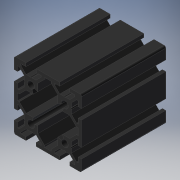
# Autodesk Inventor part: HFS5-4040-50
Saved by Autodesk Inventor 2019 (Build 230136000, 136)
## iProperties
Created: 2023-10-13
Part Number: HFS5-4040-50
Material: Generic
Catalog Web Link: www.cadenas.de
Description: NFS5-4040, NFSB5-4040, HFS5-4040, HFSB5-4040, CAF5-4040, NFSF5-4040, HFSF5-4040, HFST5-4040, HFSY5-4040-Aluminum Frames -5 Series-2 Row Groove 40 mm Square-Specified Length
Vendor: MISUMI
Document SubType Name: Modeling
Designer: psAdmin
Manufacturer: MISUMI
Mass: 24.0436 g
Surface Area: 253.98 cm^2
Volume: 24.0436 cm^3
Density: 1 g/cm^3
Appearance: PSOLRGB-175-175-175
Category: PARTsolutions
Company: MISUMI
Title: HFS5-4040-50
Author: Cadenas PARTsolutions
Comments: Aluminum Frames -5 Series-2 Row Groove 40 mm Square-Specified Length
PSOL_IDENT_0: {$CADENAS_DATA/23d-libs/misumi/metric/38_al_extrusions_blackets/5/hfs5_4040.prj},637 {VTYP=3D},{NB=H
PSOL_IDENT_1: FS5-4040-50},{LINA=HFS5-4040-50},{NN=NFS5-4040, NFSB5-4040, HFS5-4040, HFSB5-4040, CAF5-4040, NFSF5-
PSOL_IDENT_2: 4040, HFSF5-4040, HFST5-4040, HFSY5-4040},{DATE=08.05.2023 08:46:43},{GEOMDATE=23.09.2021 06:48:02},
PSOL_IDENT_3: {VERSION=},{LINEID=150},{WBVAR=L,ALT1,ALT2,ALT4,ALT5,CP5,DL5,DR5,ALT6,ALT9,ALT10,ALT11,HP6,NHL6,DL6,
PSOL_IDENT_4: NHR6,DR6,ALT7,ALT8,NH9,AH,BH,CH,DH,EH,NH10,AV,BV,CV,DV,EV,NH11,AP,BP,CP,DP,EP,ALT12,ALT13,Z,NH12,XA,
PSOL_IDENT_5: XB,XC,XD,XE,NH13,YA,YB,YC,YD,YE,ALT16,HP16,DL16,DR16,ALT17,HQ17,JLP,ALT18,HQ18,KLP,ALT20},{WBNUMERIC=
PSOL_IDENT_6: L,NH9,AH,BH,CH,DH,EH,NH10,AV,BV,CV,DV,EV,NH11,AP,BP,CP,DP,EP,NH12,XA,XB,XC,XD,XE,NH13,YA,YB,YC,YD,YE
PSOL_IDENT_7: ,HQ17,JLP,HQ18,KLP}  {NB=HFS5-4040-50},{LINA=HFS5-4040-50},{KT=DUMMY},{PN=HFS5-4040-50},{TPS=HFS5-40
PSOL_IDENT_8: 40},{MAT=A6N01SS-T5 Aluminum Alloy or 6005A-T5 Aluminum Alloy},{ST=Clear Anodize},{FRMW=40},{FRMH=40
PSOL_IDENT_9: },{FRD=4.2},{L=50},{MASS=1.28},{SA=472},{LX=8.89x10^4},{LY=8.89x10^4},{ALT1=},{M1=0},{DPL1=0},{DPR1=
PSOL_IDENT_10: 0},{ALT1PN=},{ALT2=},{ALT2ALG= '','w/o End Tapping (Insert)','LHP','with LHP (Tapping on the Left (I
PSOL_IDENT_11: nsert))','RHP','with RHP (Tapping on the Right (Insert))','HPW','with HPW (Tapping on Both Ends (Ins
PSOL_IDENT_12: ert))' },{M2=0},{DP2=0},{ALT2PN=},{ALT4=},{ALT4ALG= '', 'w/o SC (High Precision Cut)', 'SC', 'with S
PSOL_IDENT_13: C (High Precision Cut)' },{ALT4PN=},{ALT5=},{ALT5ALG= '','w/o 45 Degree Cut','1','with 45 Degree Cut'
PSOL_IDENT_14: },{CP5=},{CP5ALG= '','N/A' },{DL5=},{DL5ALG= '','N/A' },{DR5=},{DR5ALG= '','N/A' },{FRMLALT5=0},{FR
PSOL_IDENT_15: MRALT5=0},{ALT5PN=},{ALT6=},{ALT6ALG= '','w/o Fastening Location Wrench Access Hole Alterations','1'
PSOL_IDENT_16: ,'with Fastening Location Wrench Access Hole Alterations' },{ALT9=},{ALT9ALG= '','w/o Location Speci
PSOL_IDENT_17: fied Wrench Access Hole Alteratons (Horizontal)','1','with Location Specified Wrench Access Hole Alt
PSOL_IDENT_18: eratons (Horizontal)' },{ALT10=},{ALT10ALG= '','w/o Location Specified Wrench Access Hole Alteratons
PSOL_IDENT_19: (Vertical)','1','with Location Specified Wrench Access Hole Alteratons (Vertical)' },{ALT11=},{ALT1
PSOL_IDENT_20: 1ALG= '','w/o Location Specified Wrench Access Hole Alteratons (Crisscross)','1','with Location Spec
PSOL_IDENT_21: ified Wrench Access Hole Alteratons (Crisscross)' },{DD6=0.00},{DD6ALG=0},{HP6=},{HP6ALG= '','N/A' }
PSOL_IDENT_22: ,{NHL6=},{NHL6ALG= '','N/A' },{DL6=},{DL6ALG= '','N/A' },{NHR6=},{NHR6ALG= '','N/A' },{DR6=},{DR6ALG=
PSOL_IDENT_23: '','N/A' },{DD6PN=},{HL6=0},{HL6D=0},{HR6=0},{HR6D=0},{J6=0},{J6D=0},{K6=0},{K6D=0},{ALT7=},{ALT7AL
PSOL_IDENT_24: G= '','N/A' },{ALT8=},{ALT8ALG= '','N/A' },{ALT678PN=},{NH9=0},{NH9MAX=5},{NH9ALG=[0]},{AH=0.0},{AHM
PSOL_IDENT_25: IN=7},{AHMAX=45},{AHALG=[0]},{BH=0.0},{BHMIN=2},{BHMAX=47},{BHALG=[0]},{CH=0.0},{CHMIN=2},{CHMAX=49}
PSOL_IDENT_26: ,{CHALG=[0]},{DH=0.0},{DHMIN=2},{DHMAX=51},{DHALG=[0]},{EH=0.0},{EHMIN=2},{EHMAX=43},{EHALG=[0]},{NH
PSOL_IDENT_27: 10=0},{NH10MAX=5},{NH10ALG=[0]},{AV=0.0},{AVMIN=7},{AVMAX=45},{AVALG=[0]},{BV=0.0},{BVMIN=2},{BVMAX=
PSOL_IDENT_28: 47},{BVALG=[0]},{CV=0.0},{CVMIN=2},{CVMAX=49},{CVALG=[0]},{DV=0.0},{DVMIN=2},{DVMAX=51},{DVALG=[0]},
PSOL_IDENT_29: {EV=0.0},{EVMIN=2},{EVMAX=43},{EVALG=[0]},{NH11=0},{NH11MAX=5},{NH11ALG=[0]},{AP=0.0},{APMIN=7},{APM
PSOL_IDENT_30: AX=45},{APALG=[0]},{BP=0.0},{BPMIN=2},{BPMAX=47},{BPALG=[0]},{CP=0.0},{CPMIN=2},{CPMAX=49},{CPALG=[0
PSOL_IDENT_31: ]},{DP=0.0},{DPMIN=2},{DPMAX=51},{DPALG=[0]},{EP=0.0},{EPMIN=2},{EPMAX=43},{EPALG=[0]},{ALT9PN=},{AL
PSOL_IDENT_32: T10PN=},{ALT11PN=},{ALT91011PN=},{ALT12=},{ALT12ALG= '','w/o Counterbore Hole in Specified Position
PSOL_IDENT_33: (Vertical)','1','with Counterbore Hole in Specified Position (Vertical)' },{ALT13=},{ALT13ALG= '','w
PSOL_IDENT_34: /o Counterbore Hole in Specified Position (Horizontal)','1','with Counterbore Hole in Specified Posi
PSOL_IDENT_35: tion (Horizontal)' },{Z=},{ZALG= '','N/A' },{DD12=0.0},{DD112=0.0},{NH12=0},{NH12MAX=5},{NH12ALG=[0]
PSOL_IDENT_36: },{XA=0.0},{XAMIN=7},{XAMAX=45},{XAALG=[0]},{XB=0.0},{XBMIN=2},{XBMAX=47},{XBALG=[0]},{XC=0.0},{XCMI
PSOL_IDENT_37: N=2},{XCMAX=49},{XCALG=[0]},{XD=0.0},{XDMIN=2},{XDMAX=51},{XDALG=[0]},{XE=0.0},{XEMIN=2},{XEMAX=43},
PSOL_IDENT_38: {XEALG=[0]},{NH13=0},{NH13MAX=5},{NH13ALG=[0]},{YA=0.0},{YAMIN=7},{YAMAX=45},{YAALG=[0]},{YB=0.0},{Y
PSOL_IDENT_39: BMIN=2},{YBMAX=47},{YBALG=[0]},{YC=0.0},{YCMIN=2},{YCMAX=49},{YCALG=[0]},{YD=0.0},{YDMIN=2},{YDMAX=5
PSOL_IDENT_40: 1},{YDALG=[0]},{YE=0.0},{YEMIN=2},{YEMAX=43},{YEALG=[0]},{ALT12PN=},{ALT13PN=},{ALT1213PN=},{ALT16=}
PSOL_IDENT_41: ,{ALT16ALG= '','w/o M Type Hole Alteration','1','with M Type Hole Alteration' },{HP16=},{HP16ALG= ''
PSOL_IDENT_42: ,'N/A' },{DL16=},{DL16ALG= '','N/A' },{DR16=},{DR16ALG= '','N/A' },{H116=0},{D16=0.0},{ALT16PN=},{AL
PSOL_IDENT_43: T17=},{ALT17ALG= '','w/o L Type Hole Alteration (Top)','1','with L Type Hole Alteration (Top)' },{HQ
PSOL_IDENT_44: 17=0},{HQ17ALG=0},{JLP=0},{JLPMIN=4.9},{JLPMAX=0},{JLPALG=[0]},{L17=0},{D17=0.0},{ALT17PN=},{ALT18=}
PSOL_IDENT_45: ,{ALT18ALG= '','w/o L Type Hole Alteration (Bottom)','1','with L Type Hole Alteration (Bottom)' },{H
PSOL_IDENT_46: Q18=0},{HQ18ALG=0},{KLP=0},{KLPMIN=4.9},{KLPMAX=0},{KLPALG=[0]},{L18=0},{D18=0.0},{ALT18PN=},{ALT20=
PSOL_IDENT_47: },{ALT20PN=},{ERRORALT01=OK},{ERRORALT02=OK},{ERRORALT05=OK},{ERRORALT06091=OK},{ERRORALT06092=OK},{
PSOL_IDENT_48: ERRORALT06093=OK},{ERRORALT06094=OK},{ERRORALT06101=OK},{ERRORALT06102=OK},{ERRORALT06103=OK},{ERROR
PSOL_IDENT_49: ALT06104=OK},{ERRORALT06111=OK},{ERRORALT06112=OK},{ERRORALT06113=OK},{ERRORALT06114=OK},{ERRORALT06
PSOL_IDENT_50: 121=OK},{ERRORALT06122=OK},{ERRORALT06123=OK},{ERRORALT06124=OK},{ERRORALT06131=OK},{ERRORALT06132=O
PSOL_IDENT_51: K},{ERRORALT06133=OK},{ERRORALT06134=OK},{ERRORALT0616=OK},{ERRORALT06171=OK},{ERRORALT06172=OK},{ER
PSOL_IDENT_52: RORALT06173=OK},{ERRORALT06181=OK},{ERRORALT06182=OK},{ERRORALT06183=OK},{ERRORALT0911=OK},{ERRORALT
PSOL_IDENT_53: 0913=OK},{ERRORALT0916=OK},{ERRORALT0917=OK},{ERRORALT0918=OK},{ERRORALT1011=OK},{ERRORALT1012=OK},{
PSOL_IDENT_54: ERRORALT1016=OK},{ERRORALT1017=OK},{ERRORALT1018=OK},{ERRORALT1112=OK},{ERRORALT1113=OK},{ERRORALT11
PSOL_IDENT_55: 16=OK},{ERRORALT1117=OK},{ERRORALT1118=OK},{ERRORALT1216=OK},{ERRORALT1217=OK},{ERRORALT1218=OK},{ER
PSOL_IDENT_56: RORALT1316=OK},{ERRORALT1317=OK},{ERRORALT1318=OK},{ERRORALT1617=OK},{ERRORALT1618=OK},{ERRORPN=},{T
PSOL_IDENT_57: FW=0},{IDM1=4.134},{COLOR=}
NB: HFS5-4040-50
NN: NFS5-4040, NFSB5-4040, HFS5-4040, HFSB5-4040, CAF5-4040, NFSF5-4040, HFSF5-4040, HFST5-4040, HFSY5-4040
NT: Aluminum Frames -5 Series-2 Row Groove 40 mm Square-Specified Length
NBSYN: $PN.
LINA: HFS5-4040-50
CATALOG: Misumi
PN: HFS5-4040-50
TPS: HFS5-4040
MAT: A6N01SS-T5 Aluminum Alloy or 6005A-T5 Aluminum Alloy
ST: Clear Anodize
L: 50
MASS: 1.28
SA: 472
LX: 8.89x10^4
LY: 8.89x10^4
ALT1: w/o End Tapping
M1: 0
DPL1: 0
DPR1: 0
ALT2: w/o End Tapping (Insert)
M2: 0
DP2: 0
ALT4: w/o SC (High Precision Cut)
ALT5: w/o 45 Degree Cut
CP5: N/A
DL5: N/A
DR5: N/A
ALT6: w/o Fastening Location Wrench Access Hole Alterations
ALT9: w/o Location Specified Wrench Access Hole Alteratons (Horizontal)
ALT10: w/o Location Specified Wrench Access Hole Alteratons (Vertical)
ALT11: w/o Location Specified Wrench Access Hole Alteratons (Crisscross)
DD6: 0
HP6: N/A
NHL6: N/A
DL6: N/A
NHR6: N/A
DR6: N/A
HL6D: 0
HR6D: 0
J6D: 0
K6D: 0
ALT7: N/A
ALT8: N/A
NH9: 0
AH: 0
BH: 0
CH: 0
DH: 0
EH: 0
NH10: 0
AV: 0
BV: 0
CV: 0
DV: 0
EV: 0
NH11: 0
AP: 0
BP: 0
CP: 0
DP: 0
EP: 0
ALT12: w/o Counterbore Hole in Specified Position (Vertical)
ALT13: w/o Counterbore Hole in Specified Position (Horizontal)
Z: N/A
DD12: 0
DD112: 0
NH12: 0
XA: 0
XB: 0
XC: 0
XD: 0
XE: 0
NH13: 0
YA: 0
YB: 0
YC: 0
YD: 0
YE: 0
ALT16: w/o M Type Hole Alteration
HP16: N/A
DL16: N/A
DR16: N/A
H116: 0
D16: 0
ALT17: w/o L Type Hole Alteration (Top)
HQ17: 0
JLP: 0
D17: 0
ALT18: w/o L Type Hole Alteration (Bottom)
HQ18: 0
KLP: 0
D18: 0
ALT20: w/o CW (End Face C Chamfering)
SUPPLIER: MISUMI
ARTICLENO: HFS5-4040-50
BOMINFO: HFS5-4040-50
CREATOR: CADENAS GmbH
Autodesk Inventor part; units mm, degrees
sketch "Sketch_1" plane through (0, 0, 0) normal (0, 0, 1) x (1, 0, 0)
  line L0 (-20, -7) -> (-18, -7)
  line L1 (-18, -7) -> (-18, -4)
  line L2 (-18, -4) -> (-17.0607, -4)
  line L3 (-17.0607, -4) -> (-14, -7.0607)
  line L4 (-14, -7.0607) -> (-14, -9.4804)
  line L5 (-14, -9.4804) -> (-13.7, -10)
  line L6 (-13.7, -10) -> (-14, -10.5196)
  line L7 (-14, -10.5196) -> (-14, -12.9393)
  line L8 (-14, -12.9393) -> (-17.0607, -16)
  line L9 (-17.0607, -16) -> (-18, -16)
  line L10 (-18, -16) -> (-18, -13)
  line L11 (-18, -13) -> (-20, -13)
  line L12 (-20, -13) -> (-20, -19)
  arc A0 (-20, -19) -> (-19, -20) centre (-19, -19) ccw
  line L13 (-19, -20) -> (-13, -20)
  line L14 (-13, -20) -> (-13, -18)
  line L15 (-13, -18) -> (-16, -18)
  line L16 (-16, -18) -> (-16, -17.0607)
  line L17 (-16, -17.0607) -> (-12.9393, -14)
  line L18 (-12.9393, -14) -> (-10.5196, -14)
  line L19 (-10.5196, -14) -> (-10, -13.7)
  line L20 (-10, -13.7) -> (-9.4804, -14)
  line L21 (-9.4804, -14) -> (-7.0607, -14)
  line L22 (-7.0607, -14) -> (-4, -17.0607)
  line L23 (-4, -17.0607) -> (-4, -18)
  line L24 (-4, -18) -> (-7, -18)
  line L25 (-7, -18) -> (-7, -20)
  line L26 (-7, -20) -> (7, -20)
  line L27 (7, -20) -> (7, -18)
  line L28 (7, -18) -> (4, -18)
  line L29 (4, -18) -> (4, -17.0607)
  line L30 (4, -17.0607) -> (7.0607, -14)
  line L31 (7.0607, -14) -> (9.4804, -14)
  line L32 (9.4804, -14) -> (10, -13.7)
  line L33 (10, -13.7) -> (10.5196, -14)
  line L34 (10.5196, -14) -> (12.9393, -14)
  line L35 (12.9393, -14) -> (16, -17.0607)
  line L36 (16, -17.0607) -> (16, -18)
  line L37 (16, -18) -> (13, -18)
  line L38 (13, -18) -> (13, -20)
  line L39 (13, -20) -> (19, -20)
  arc A1 (19, -20) -> (20, -19) centre (19, -19) ccw
  line L40 (20, -19) -> (20, -13)
  line L41 (20, -13) -> (18, -13)
  line L42 (18, -13) -> (18, -16)
  line L43 (18, -16) -> (17.0607, -16)
  line L44 (17.0607, -16) -> (14, -12.9393)
  line L45 (14, -12.9393) -> (14, -10.5196)
  line L46 (14, -10.5196) -> (13.7, -10)
  line L47 (13.7, -10) -> (14, -9.4804)
  line L48 (14, -9.4804) -> (14, -7.0607)
  line L49 (14, -7.0607) -> (17.0607, -4)
  line L50 (17.0607, -4) -> (18, -4)
  line L51 (18, -4) -> (18, -7)
  line L52 (18, -7) -> (20, -7)
  line L53 (20, -7) -> (20, 7)
  line L54 (20, 7) -> (18, 7)
  line L55 (18, 7) -> (18, 4)
  line L56 (18, 4) -> (17.0607, 4)
  line L57 (17.0607, 4) -> (14, 7.0607)
  line L58 (14, 7.0607) -> (14, 9.4804)
  line L59 (14, 9.4804) -> (13.7, 10)
  line L60 (13.7, 10) -> (14, 10.5196)
  line L61 (14, 10.5196) -> (14, 12.9393)
  line L62 (14, 12.9393) -> (17.0607, 16)
  line L63 (17.0607, 16) -> (18, 16)
  line L64 (18, 16) -> (18, 13)
  line L65 (18, 13) -> (20, 13)
  line L66 (20, 13) -> (20, 19)
  arc A2 (20, 19) -> (19, 20) centre (19, 19) ccw
  line L67 (19, 20) -> (13, 20)
  line L68 (13, 20) -> (13, 18)
  line L69 (13, 18) -> (16, 18)
  line L70 (16, 18) -> (16, 17.0607)
  line L71 (16, 17.0607) -> (12.9393, 14)
  line L72 (12.9393, 14) -> (10.5196, 14)
  line L73 (10.5196, 14) -> (10, 13.7)
  line L74 (10, 13.7) -> (9.4804, 14)
  line L75 (9.4804, 14) -> (7.0607, 14)
  line L76 (7.0607, 14) -> (4, 17.0607)
  line L77 (4, 17.0607) -> (4, 18)
  line L78 (4, 18) -> (7, 18)
  line L79 (7, 18) -> (7, 20)
  line L80 (7, 20) -> (-7, 20)
  line L81 (-7, 20) -> (-7, 18)
  line L82 (-7, 18) -> (-4, 18)
  line L83 (-4, 18) -> (-4, 17.0607)
  line L84 (-4, 17.0607) -> (-7.0607, 14)
  line L85 (-7.0607, 14) -> (-9.4804, 14)
  line L86 (-9.4804, 14) -> (-10, 13.7)
  line L87 (-10, 13.7) -> (-10.5196, 14)
  line L88 (-10.5196, 14) -> (-12.9393, 14)
  line L89 (-12.9393, 14) -> (-16, 17.0607)
  line L90 (-16, 17.0607) -> (-16, 18)
  line L91 (-16, 18) -> (-13, 18)
  line L92 (-13, 18) -> (-13, 20)
  line L93 (-13, 20) -> (-19, 20)
  arc A3 (-19, 20) -> (-20, 19) centre (-19, 19) ccw
  line L94 (-20, 19) -> (-20, 13)
  line L95 (-20, 13) -> (-18, 13)
  line L96 (-18, 13) -> (-18, 16)
  line L97 (-18, 16) -> (-17.0607, 16)
  line L98 (-17.0607, 16) -> (-14, 12.9393)
  line L99 (-14, 12.9393) -> (-14, 10.5196)
  line L100 (-14, 10.5196) -> (-13.7, 10)
  line L101 (-13.7, 10) -> (-14, 9.4804)
  line L102 (-14, 9.4804) -> (-14, 7.0607)
  line L103 (-14, 7.0607) -> (-17.0607, 4)
  line L104 (-17.0607, 4) -> (-18, 4)
  line L105 (-18, 4) -> (-18, 7)
  line L106 (-18, 7) -> (-20, 7)
  line L107 (-20, 7) -> (-20, -7)
  constraints: 216 end point, 8 point on circle, 4 centre point
extrude "Extrusion1" add sketch "Sketch_1" against normal blind 50
sketch "Sketch_130" plane through (0, 0, 0) normal (0, 0, 1) x (1, 0, 0)
  line L0 (-18, 2) -> (-18, -2)
  line L1 (-18, -2) -> (-16.9393, -2)
  line L2 (-16.9393, -2) -> (-12.9393, -6)
  line L3 (-12.9393, -6) -> (-8.6667, -6)
  line L4 (-8.6667, -6) -> (-9.3359, -8.0078)
  arc A0 (-9.3359, -8.0078) -> (-8.0078, -9.3359) centre (-10, -10) ccw
  line L5 (-8.0078, -9.3359) -> (-6, -8.6667)
  line L6 (-6, -8.6667) -> (-6, -12.9393)
  line L7 (-6, -12.9393) -> (-2, -16.9393)
  line L8 (-2, -16.9393) -> (-2, -18)
  line L9 (-2, -18) -> (2, -18)
  line L10 (2, -18) -> (2, -16.9393)
  line L11 (2, -16.9393) -> (6, -12.9393)
  line L12 (6, -12.9393) -> (6, -8.6667)
  line L13 (6, -8.6667) -> (8.0078, -9.3359)
  arc A1 (8.0078, -9.3359) -> (9.3359, -8.0078) centre (10, -10) ccw
  line L14 (9.3359, -8.0078) -> (8.6667, -6)
  line L15 (8.6667, -6) -> (12.9393, -6)
  line L16 (12.9393, -6) -> (16.9393, -2)
  line L17 (16.9393, -2) -> (18, -2)
  line L18 (18, -2) -> (18, 2)
  line L19 (18, 2) -> (16.9393, 2)
  line L20 (16.9393, 2) -> (12.9393, 6)
  line L21 (12.9393, 6) -> (8.6667, 6)
  line L22 (8.6667, 6) -> (9.3359, 8.0078)
  arc A2 (9.3359, 8.0078) -> (8.0078, 9.3359) centre (10, 10) ccw
  line L23 (8.0078, 9.3359) -> (6, 8.6667)
  line L24 (6, 8.6667) -> (6, 12.9393)
  line L25 (6, 12.9393) -> (2, 16.9393)
  line L26 (2, 16.9393) -> (2, 18)
  line L27 (2, 18) -> (-2, 18)
  line L28 (-2, 18) -> (-2, 16.9393)
  line L29 (-2, 16.9393) -> (-6, 12.9393)
  line L30 (-6, 12.9393) -> (-6, 8.6667)
  line L31 (-6, 8.6667) -> (-8.0078, 9.3359)
  arc A3 (-8.0078, 9.3359) -> (-9.3359, 8.0078) centre (-10, 10) ccw
  line L32 (-9.3359, 8.0078) -> (-8.6667, 6)
  line L33 (-8.6667, 6) -> (-12.9393, 6)
  line L34 (-12.9393, 6) -> (-16.9393, 2)
  line L35 (-16.9393, 2) -> (-18, 2)
  constraints: 72 end point, 8 point on circle, 4 centre point
extrude "Extrusion2" cut sketch "Sketch_130" against normal blind 50
ref_plane "C1_XY" through (0, 0, 0) normal (0, 0, 1) x (1, 0, 0)
ref_plane "C1_YZ" through (0, 0, 0) normal (1, 0, 0) x (0, 1, 0)
ref_plane "C1_ZX" through (0, 0, 0) normal (0, 1, 0) x (0, 0, 1)
ref_plane "to_frame_cap1_XY" through (0, 0, 0) normal (0, 0, 1) x (1, 0, 0)
ref_plane "to_frame_cap1_YZ" through (0, 0, 0) normal (1, 0, 0) x (0, 1, 0)
ref_plane "to_frame_cap1_ZX" through (0, 0, 0) normal (0, 1, 0) x (0, 0, 1)
ref_plane "to_frame_cap2_XY" through (0, 0, -50) normal (0, 0, -1) x (1, 0, 0)
ref_plane "to_frame_cap2_YZ" through (0, 0, -50) normal (1, 0, 0) x (0, -1, 0)
ref_plane "to_frame_cap2_ZX" through (0, 0, -50) normal (0, -1, 0) x (0, 0, -1)
body "Solid1"
